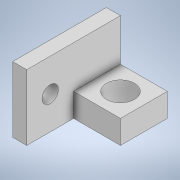
# Autodesk Inventor part: IRSensorMount
Saved by Autodesk Inventor 2020.3 (Build 243373000, 373)
## iProperties
Created: 2020-08-18
Part Number: IRSensorMount
Material: Generic
Document SubType Name: Modeling
Designer: joesp
Density: 1 g/cm^3
Appearance: Default
Author: joesp
Autodesk Inventor part; units mm, degrees
ref_plane "YZ Plane" through (0, 0, 0) normal (1, 0, 0) x (0, 1, 0)
ref_plane "XZ Plane" through (0, 0, 0) normal (0, 1, 0) x (-1, 0, 0)
ref_plane "XY Plane" through (0, 0, 0) normal (0, 0, 1) x (1, 0, 0)
sketch "Sketch2" plane through (0, 0, 0) normal (1, 0, 0) x (0, 1, 0)
  line L0 (0, 0) -> (14, 0)
  line L1 (14, 0) -> (14, -20)
  line L2 (14, -20) -> (0, -20)
  line L3 (0, -20) -> (0, 0)
  circle A0 centre (7, -5) radius 1.75
  circle A1 centre (7, -5) radius 3.5 construction
  point P0 (0, -10)
  point P1 (7, -20)
  dimension "d11" = 20
  dimension "d24" = 14
  dimension "d27" = 3.5
  dimension "d28" = 7
  dimension "d29" = 5
  constraints: 8 end point, 2 centre point, 2 midpoint, 2 perpendicular, 1 coincident, 1 horizontal, 1 vertical, 1 vertical alignment
  measures "d11" distance of L0.end L1.end
  measures "d24" distance of L1.end L2.end
  measures "d27" diameter of A0
  measures "d28" diameter of A1
  measures "d29" distance from line of L0 A0.centre
extrude "Extrusion1" add sketch "Sketch2" along normal blind 3
sketch "Sketch3" plane through (3, 0, 0) normal (1, 0, 0) x (0, 0, -1)
  line L0 (0, 0) -> (20, 0) projected
  line L1 (20, 0) -> (10, 0)
  line L2 (10, 0) -> (10, 5)
  line L3 (10, 5) -> (20, 5)
  line L4 (20, 5) -> (20, 0)
  point P0 (10, 0)
  dimension "d12" = 5
  dimension "d13" = 10
  constraints: 8 end point, 2 parallel, 1 horizontal, 1 perpendicular
  measures "d12" distance of L1.end L2.end
  measures "d13" distance of L2.end L3.end
extrude "Extrusion2" add sketch "Sketch3" along normal blind 10
sketch "Sketch4" plane through (3, 5, -10) normal (0, 1, 0) x (1, 0, 0)
  circle A0 centre (5, 5) radius 3
  line L0 (10, 10) -> (10, 0) projected
  point P0 (-3, -10)
  point P1 (10, 5)
  dimension "d16" = 6
  dimension "d17" = 5
  constraints: 1 centre point, 1 horizontal alignment, 1 midpoint
  measures "d16" diameter of A0
  measures "d17" distance from line of L0 A0.centre
extrude "Extrusion3" cut sketch "Sketch4" against normal through all
body "Solid1"
